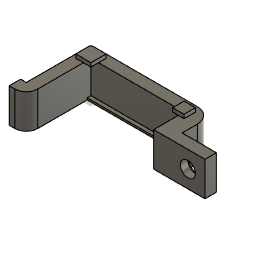
StepperMount v10 (Autodesk Fusion 360 design; units mm, degrees)
Autodesk Fusion 360 part; units mm, degrees
note: some values were not read from the file. Set by a fixed rule: which sketch regions a step uses.
sketch "草图1" plane through (0, 0, 0) normal (0, 1, 0) x (1, 0, 0)
  line L0 (12, 9) -> (36.5, 9)
  line L1 (37, 12) -> (13, 12)
  line L2 (9, 8) -> (9, -5)
  line L3 (12, 9) -> (12, -5)
  arc A0 (9, -8) -> (12, -5) centre (9, -5) ccw
  arc A1 (13, 12) -> (9, 8) centre (13, 8) ccw
  line L4 (9, -5) -> (8.5, -5)
  line L5 (8.5, -8) -> (9, -8)
  line L6 (38, 1) -> (50, 1)
  line L7 (50, 1) -> (50, 4)
  line L8 (50, 4) -> (41, 4)
  line L9 (37, 12) -> (37, 12)
  line L10 (41, 8) -> (41, 4)
  arc A2 (41, 8) -> (37, 12) centre (37, 8) ccw
  line L11 (8.5, -5) -> (7.5, -5)
  line L12 (7.5, -5) -> (7.5, -8)
  line L13 (7.5, -8) -> (8.5, -8)
  line L14 (38, 1) -> (36.5, 1)
  line L15 (36.5, 1) -> (36.5, 9)
  dimension "d21" = 3
  dimension "d22" = 4
  dimension "d30" = 4
  constraint perpendicular L0 L3
  constraint tangent L3 A0
  constraint tangent L1 A1
  constraint tangent L2 A1
  constraint perpendicular L2 L4
  constraint tangent A0 L5
  constraint perpendicular L8 L10
  constraint tangent L10 A2
  constraint perpendicular L2 L11
  constraint perpendicular L11 L12
  constraint perpendicular L12 L13
  constraint perpendicular L14 L15
  measures "d21" radius of A0
  measures "d22" radius of A1
  measures "d30" radius of A2
extrude "拉伸1" add sketch "草图1" along normal blind 10
move_body "移动1" bodies 1 to x (1, 0, 0) y (0, 1, 0) z (0, 0, 1) at (-25, 0, 0)
extrude "拉伸2" cut 1 faces at (13, 10, -4.6667) along direction (0, -1, 0) blind 1
hole "孔5" at (20.5, 4.5, -4) direction (0, 0, 1) diameter 4 depth 4 tip angle 180 countersink diameter 6 countersink angle 90
sketch "草图4" plane through (0, 9, 0) normal (0, 1, 0) x (-1, 0, 0)
  arc A0 (-16, -8) -> (-12, -12) centre (-12, -8) ccw
  line L0 (-12, -12) -> (12, -12)
  arc A1 (12, -12) -> (16, -8) centre (12, -8) ccw
  line L1 (16, -8) -> (16, 5)
  line L2 (16, 5) -> (17.5, 5)
  line L3 (17.5, 5) -> (17.5, 8)
  line L4 (17.5, 8) -> (16, 8)
  arc A2 (16, 8) -> (13, 5) centre (16, 5) ccw
  line L5 (13, 5) -> (13, -9)
  line L6 (13, -9) -> (-11.5, -9)
  line L7 (-11.5, -1) -> (-25, -1)
  line L8 (-25, -1) -> (-25, -4)
  line L9 (-25, -4) -> (-16, -4)
  line L10 (-16, -4) -> (-16, -8)
  line L11 (13, 0) -> (7, 0)
  line L12 (7, 0) -> (7, -4.5)
  circle A3 centre (7, -4.5) radius 3.8
  line L13 (11, -7) -> (15, -7)
  line L14 (15, -7) -> (15, -11)
  line L15 (15, -11) -> (11, -11)
  line L16 (11, -11) -> (11, -7)
  line L17 (-10, -7.5) -> (-13, -7.5)
  line L18 (-13, -7.5) -> (-13, -10.5)
  line L19 (-13, -10.5) -> (-10, -10.5)
  line L20 (-10, -10.5) -> (-10, -7.5)
  line L21 (-11.5, -9) -> (-11.5, -1)
  constraint coincident L5 L11.start
  constraint perpendicular L5 L11
  constraint perpendicular L6 L12
  constraint coincident L12.end A3.centre
  constraint horizontal L13
  constraint vertical L14
  constraint horizontal L15
  constraint vertical L16
  constraint horizontal L17
  constraint vertical L18
  constraint horizontal L19
  constraint vertical L20
extrude "拉伸3" add sketch "草图4" along normal blind 1 contours A1 L5 L6 L13 L14 L15 L16 | L5 L6 L13 L16
extrude "拉伸4" add sketch "草图4" along normal blind 1 contours L6 L17 L18 L19 L20 L21 | L6 L17 L20 L21
sketch "草图5" plane through (0, 0, 0) normal (0, -1, 0) x (1, 0, 0)
  line L0 (25, -1) -> (11.5, -1)
  line L1 (11.5, -1) -> (11.5, -9)
  line L2 (11.5, -9) -> (-13, -9)
  line L3 (-13, -9) -> (-13, 5)
  arc A0 (-13, 5) -> (-16, 8) centre (-16, 5) ccw
  line L4 (-16, 8) -> (-17.5, 8)
  line L5 (-17.5, 8) -> (-17.5, 5)
  line L6 (-17.5, 5) -> (-16, 5)
  line L7 (-16, 5) -> (-16, -8)
  arc A1 (-16, -8) -> (-12, -12) centre (-12, -8) ccw
  line L8 (-12, -12) -> (12, -12)
  arc A2 (12, -12) -> (16, -8) centre (12, -8) ccw
  line L9 (16, -8) -> (16, -4)
  line L10 (16, -4) -> (25, -4)
  line L11 (25, -4) -> (25, -1)
  line L12 (-13, -9) -> (11.5, -9)
  line L13 (11.5, -9) -> (11.5, -8)
  line L14 (11.5, -8) -> (-13, -8)
  line L15 (-13, -8) -> (-13, -9)
  dimension "d43" = 1
  constraint horizontal L12
  constraint vertical L13
  constraint horizontal L14
  constraint vertical L15
  constraint coincident L2.end L3.start
  measures "d43" distance of L2.end L14.end
extrude "拉伸5" add sketch "草图5" against normal blind 0.5
